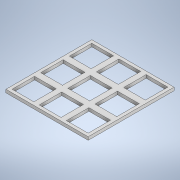
# Autodesk Inventor part: Keyframe3by3
Saved by Autodesk Inventor 2021 (Build 250183000, 183)
## iProperties
Created: 2021-04-29
Part Number: Keyframe3by3
Material: Generic
Document SubType Name: Modeling
Designer: email
Density: 1 g/cm^3
Appearance: Default
Author: email
Autodesk Inventor part; units mm, degrees
ref_plane "YZ Plane" through (0, 0, 0) normal (1, 0, 0) x (0, 1, 0)
ref_plane "XZ Plane" through (0, 0, 0) normal (0, 1, 0) x (-1, 0, 0)
ref_plane "XY Plane" through (0, 0, 0) normal (0, 0, 1) x (1, 0, 0)
sketch "Sketch1" plane through (0, 0, 0) normal (0, 1, 0) x (-1, 0, 0)
  line L0 (-24.625, 24.95) -> (-24.625, -24.95)
  line L1 (24.625, 24.95) -> (-24.625, -24.95) construction
  line L2 (-24.625, 24.95) -> (24.625, -24.95) construction
  line L3 (-24.625, 22.95) -> (-22.625, 22.95) construction
  line L4 (-22.625, 24.95) -> (-22.625, 22.95) construction
  line L5 (-22.625, 22.95) -> (-8.575, 22.95)
  line L6 (-8.575, 22.95) -> (-8.575, 8.45)
  line L7 (-8.575, 8.45) -> (-22.625, 8.45)
  line L8 (-22.625, 8.45) -> (-22.625, 22.95)
  line L9 (-22.625, 8.45) -> (-22.625, 4.45) construction
  line L10 (-22.625, 4.45) -> (-8.575, 4.45)
  line L11 (-8.575, 4.45) -> (-8.575, -10.05)
  line L12 (-8.575, -10.05) -> (-22.625, -10.05)
  line L13 (-22.625, -10.05) -> (-22.625, 4.45)
  line L14 (-22.625, -10.05) -> (-22.625, -14.05) construction
  line L15 (-22.625, -14.05) -> (-8.575, -14.05)
  line L16 (-8.575, -14.05) -> (-8.575, -28.55)
  line L17 (-8.575, -28.55) -> (-22.625, -28.55)
  line L18 (-22.625, -28.55) -> (-22.625, -14.05)
  line L19 (-8.575, 22.95) -> (-5.075, 22.95) construction
  line L20 (-5.075, 22.95) -> (8.975, 22.95)
  line L21 (8.975, 22.95) -> (8.975, 8.45)
  line L22 (8.975, 8.45) -> (-5.075, 8.45)
  line L23 (-5.075, 8.45) -> (-5.075, 22.95)
  line L24 (-5.075, 8.45) -> (-5.075, 4.45)
  line L25 (-5.075, 4.45) -> (8.975, 4.45)
  line L26 (8.975, 4.45) -> (8.975, -10.05)
  line L27 (8.975, -10.05) -> (-5.075, -10.05)
  line L28 (-5.075, -10.05) -> (-5.075, 4.45)
  line L29 (-5.075, -10.05) -> (-5.075, -14.05) construction
  line L30 (-5.075, -14.05) -> (8.975, -14.05)
  line L31 (8.975, -14.05) -> (8.975, -28.55)
  line L32 (8.975, -28.55) -> (-5.075, -28.55)
  line L33 (-5.075, -28.55) -> (-5.075, -14.05)
  line L34 (8.975, 22.95) -> (12.475, 22.95) construction
  line L35 (12.475, 22.95) -> (26.525, 22.95)
  line L36 (26.525, 22.95) -> (26.525, 8.45)
  line L37 (26.525, 8.45) -> (12.475, 8.45)
  line L38 (12.475, 8.45) -> (12.475, 22.95)
  line L39 (8.975, 4.45) -> (12.475, 4.45) construction
  line L40 (12.475, 4.45) -> (26.525, 4.45)
  line L41 (26.525, 4.45) -> (26.525, -10.05)
  line L42 (26.525, -10.05) -> (12.475, -10.05)
  line L43 (12.475, -10.05) -> (12.475, 4.45)
  line L44 (12.475, -10.05) -> (12.475, -14.05) construction
  line L45 (12.475, -14.05) -> (26.525, -14.05)
  line L46 (26.525, -14.05) -> (26.525, -28.55)
  line L47 (26.525, -28.55) -> (12.475, -28.55)
  line L48 (12.475, -28.55) -> (12.475, -14.05)
  line L49 (-22.625, 24.95) -> (-24.625, 24.95)
  line L50 (-24.625, 24.95) -> (28.525, 24.95)
  line L51 (28.525, 24.95) -> (28.525, -30.55)
  line L52 (28.525, -30.55) -> (-24.625, -30.55)
  line L53 (-24.625, -30.55) -> (-24.625, 24.95)
  point P0 (0, 0)
  dimension "d3" = 2
  dimension "d4" = 14.5
  dimension "d5" = 14.05
  dimension "d6" = 4
  dimension "d7" = 14.5
  dimension "d8" = 14.05
  dimension "d9" = 4
  dimension "d10" = 14.5
  dimension "d11" = 14.05
  dimension "d12" = 2
  dimension "d13" = 3.5
  dimension "d14" = 14.5
  dimension "d15" = 14.05
  dimension "d16" = 4
  dimension "d17" = 14.5
  dimension "d18" = 14.05
  dimension "d19" = 4
  dimension "d20" = 14.5
  dimension "d21" = 3.5
  dimension "d22" = 14.05
  dimension "d23" = 3.5
  dimension "d24" = 14.5
  dimension "d25" = 4
  dimension "d26" = 14.5
  dimension "d27" = 55.5
  dimension "d28" = 53.15
  dimension "d29" = 14.05
  dimension "d32" = 14.5
  constraints: 108 end point, 20 parallel, 13 horizontal, 11 perpendicular, 6 vertical, 2 midpoint, 1 point on line
  measures "d3" distance of L3.start L3.end
  measures "d4" distance of L5.end L6.end
  measures "d5" distance of L6.end L7.end
  measures "d6" distance of L7.end L9.end
  measures "d7" distance of L10.end L11.end
  measures "d8" distance of L11.end L12.end
  measures "d9" distance of L12.end L14.end
  measures "d10" distance of L15.end L16.end
  measures "d11" distance of L16.end L17.end
  measures "d12" distance of L4.start L3.end
  measures "d13" distance of L5.end L19.end
  measures "d14" distance of L20.end L21.end
  measures "d15" distance of L21.end L22.end
  measures "d16" distance of L22.end L24.end
  measures "d17" distance of L25.end L26.end
  measures "d18" distance of L26.end L27.end
  measures "d19" distance of L27.end L29.end
  measures "d20" distance of L30.end L31.end
  measures "d21" distance of L20.end L34.end
  measures "d22" distance of L36.end L37.end
  measures "d23" distance of L25.end L39.end
  measures "d24" distance of L40.end L41.end
  measures "d25" distance of L42.end L44.end
  measures "d26" distance of L45.end L46.end
  measures "d27" distance of L50.end L51.end
  measures "d28" distance of L51.end L52.end
  measures "d29" distance of L41.end L42.end
  measures "d32" distance of L37.end L34.end
extrude "Extrusion1" add sketch "Sketch1" along normal blind 2
body "Solid1"
